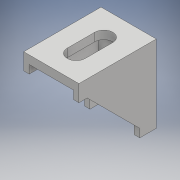
# Autodesk Inventor part: Ke NHOM 28x28x20
Saved by Autodesk Inventor 2017 (Build 210142000, 142)
## iProperties
Created: 2019-04-30
Part Number: Ke NHOM 28x28x20
Material: Generic
Document SubType Name: Modeling
Designer: Admin
Density: 1 g/cm^3
Appearance: Default
Author: Admin
Autodesk Inventor part; units mm, degrees
ref_plane "YZ Plane" through (0, 0, 0) normal (1, 0, 0) x (0, 1, 0)
ref_plane "XZ Plane" through (0, 0, 0) normal (0, 1, 0) x (-1, 0, 0)
ref_plane "XY Plane" through (0, 0, 0) normal (0, 0, 1) x (1, 0, 0)
sketch "Sketch1" plane through (0, 0, 0) normal (0, 1, 0) x (-1, 0, 0)
  line L0 (10, -14) -> (-10, -14)
  line L1 (-10, -14) -> (-10, 14)
  line L2 (-10, 14) -> (10, 14)
  line L3 (10, 14) -> (10, -14)
  line L4 (10, -14) -> (-10, 14) construction
  line L5 (-10, -14) -> (10, 14) construction
  point P0 (0, 0)
  dimension "d0" = 20
  dimension "d1" = 28
  constraints: 12 end point, 2 midpoint, 2 parallel, 1 horizontal, 1 perpendicular
  measures "d0" distance of L1.end L2.end
  measures "d1" distance of L0.end L1.end
extrude "Extrusion1" add sketch "Sketch1" along normal blind 3
sketch "Sketch2" plane through (0, 0, 0) normal (0, -1, 0) x (1, 0, 0)
  line L0 (-10, 14) -> (10, 14) projected
  line L1 (-10, 14) -> (10, 14)
  line L2 (10, 14) -> (10, 11)
  line L3 (10, 11) -> (-10, 11)
  line L4 (-10, 11) -> (-10, 14)
  point P0 (0, 0)
  dimension "d4" = 20
  dimension "d5" = 3
  constraints: 8 end point, 2 parallel, 1 horizontal, 1 perpendicular
  measures "d4" distance of L2.end L3.end
  measures "d5" distance of L1.end L2.end
extrude "Extrusion2" add sketch "Sketch2" along normal blind 25
sketch "Sketch3" plane through (10, 0, -14) normal (1, 0, 0) x (0, 0, -1)
  line L0 (-25, 0) -> (-25, -25) projected
  line L1 (0, 0) -> (-25, 0) projected
  line L2 (0, 0) -> (-25, 0)
  line L3 (-25, 0) -> (-25, -25)
  line L4 (-25, -25) -> (-22, -25)
  line L5 (-22, -25) -> (-22, -22)
  line L6 (0, 0) -> (0, 3) projected
  line L7 (0, 0) -> (0, -3)
  line L8 (0, -3) -> (-3, -3)
  line L9 (-3, -3) -> (-22, -22)
  point P0 (-14, 0)
  dimension "d8" = 3
  dimension "d9" = 3
  dimension "d10" = 3
  dimension "d11" = 3
  constraints: 14 end point, 3 perpendicular, 1 collinear, 1 horizontal, 1 vertical
  measures "d8" distance of L0.end L4.end
  measures "d9" distance of L4.end L5.end
  measures "d10" distance of L1.start L7.end
  measures "d11" distance of L7.end L8.end
extrude "Extrusion3" add sketch "Sketch3" against normal blind 2
mirror "Mirror1" about plane through (0, 0, 0) normal (1, 0, 0) of "Extrusion3"
sketch "Sketch4" plane through (-10, 3, 14) normal (0, 0, 1) x (1, 0, 0)
  line L0 (2, -28) -> (18, -28) projected
  line L1 (6.75, -9) -> (13.25, -9)
  line L2 (13.25, -9) -> (13.25, -19)
  line L3 (13.25, -19) -> (6.75, -19)
  line L4 (6.75, -19) -> (6.75, -9)
  line L5 (6.75, -9) -> (13.25, -19) construction
  line L6 (13.25, -9) -> (6.75, -19) construction
  arc A0 (13.25, -9) -> (6.75, -9) centre (10, -9) ccw
  arc A1 (6.75, -19) -> (13.25, -19) centre (10, -19) ccw
  point P0 (10, -3)
  point P1 (10, -14)
  dimension "d14" = 6.5
  dimension "d15" = 10
  constraints: 12 end point, 4 midpoint, 4 point on circle, 2 centre point, 2 parallel, 1 horizontal, 1 perpendicular
  measures "d14" distance of L2.end L3.end
  measures "d15" distance of L1.end L2.end
extrude "Extrusion4" cut sketch "Sketch4" against normal through all
sketch "Sketch5" plane through (0, 3, 0) normal (0, 1, 0) x (1, 0, 0)
  line L0 (3.25, -5) -> (-3.25, -5)
  line L1 (-3.25, -5) -> (-3.25, 5)
  line L2 (-3.25, 5) -> (3.25, 5)
  line L3 (3.25, 5) -> (3.25, -5)
  line L4 (3.25, -5) -> (-3.25, 5) construction
  line L5 (-3.25, -5) -> (3.25, 5) construction
  arc A0 (-3.25, -5) -> (3.25, -5) centre (0, -5) ccw
  arc A1 (3.25, 5) -> (-3.25, 5) centre (0, 5) ccw
  point P0 (0, 0)
  dimension "d18" = 6.5
  dimension "d19" = 10
  constraints: 12 end point, 4 midpoint, 4 point on circle, 2 centre point, 2 parallel, 1 horizontal, 1 perpendicular
  measures "d18" distance of L1.end L2.end
  measures "d19" distance of L0.end L1.end
extrude "Extrusion5" cut sketch "Sketch5" against normal through all
body "Solid1"
